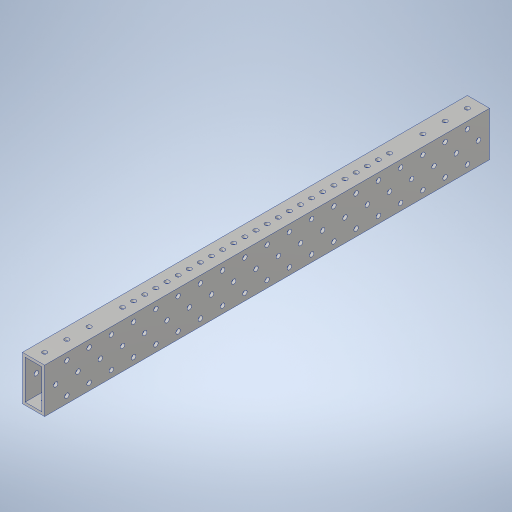
# Autodesk Inventor part: DB1-001
Saved by Autodesk Inventor 2023.4 (Build 274418000, 418)
## iProperties
RuleStatus: InUse
Created: 2025-01-07
Part Number: DB1-001
Material: Aluminum 6061
Document SubType Name: Modeling
Designer: mavericks
Mass: 304.185 g
Surface Area: 718.547 cm^2
Volume: 112.661 cm^3
Density: 2.7 g/cm^3
Appearance: Aluminum - Flat
AfterDocNew0: SHOW
AfterDocOpen0: SHOW
Author: mavericks
Autodesk Inventor part; units mm, degrees
ref_plane "YZ Plane" through (0, 0, 0) normal (1, 0, 0) x (0, 1, 0)
ref_plane "XZ Plane" through (0, 0, 0) normal (0, 1, 0) x (-1, 0, 0)
ref_plane "XY Plane" through (0, 0, 0) normal (0, 0, 1) x (1, 0, 0)
sketch "Sketch1" plane through (0, 0, 0) normal (0, 0, 1) x (1, 0, 0)
  line L0 (-12.7, -25.4) -> (12.7, -25.4)
  line L1 (12.7, -25.4) -> (12.7, 25.4)
  line L2 (12.7, 25.4) -> (-12.7, 25.4)
  line L3 (-12.7, 25.4) -> (-12.7, -25.4)
  line L4 (-12.7, -25.4) -> (12.7, 25.4) construction
  line L5 (12.7, -25.4) -> (-12.7, 25.4) construction
  line L6 (-9.525, 22.225) -> (9.525, 22.225)
  line L7 (9.525, 22.225) -> (9.525, -22.225)
  line L8 (9.525, -22.225) -> (-9.525, -22.225)
  line L9 (-9.525, -22.225) -> (-9.525, 22.225)
  point P0 (0, 0)
  dimension "width" = 25.4
  dimension "height" = 50.8
  dimension "thickness" = 3.175
  constraints: 20 end point, 4 parallel, 2 midpoint, 2 perpendicular, 1 horizontal, 3 other
  measures "width" distance of L2.end L1.end
  measures "height" distance of L1.end L0.end
  measures "thickness" distance between parallel lines of L2 L6
extrude "Extrusion1" add sketch "Sketch1" along normal mid plane 508
sketch "Sketch2" plane through (-12.7, 25.4, 254) normal (0, 1, 0) x (1, 0, 0)
  line L0 (25.4, 0) -> (0, 0) projected
  line L1 (12.7, 254) -> (0, 254) construction
  line L2 (0, 0) -> (0, 508) projected
  line L3 (12.7, 266.7) -> (12.7, 241.3) construction
  line L4 (12.7, 254) -> (12.7, 228.6) construction
  line L5 (12.7, 241.3) -> (12.7, 215.9) construction
  line L6 (12.7, 228.6) -> (12.7, 203.2) construction
  line L7 (12.7, 215.9) -> (12.7, 190.5) construction
  line L8 (12.7, 203.2) -> (12.7, 177.8) construction
  line L9 (12.7, 190.5) -> (12.7, 165.1) construction
  line L10 (12.7, 177.8) -> (12.7, 152.4) construction
  line L11 (12.7, 165.1) -> (12.7, 139.7) construction
  line L12 (12.7, 152.4) -> (12.7, 127) construction
  line L13 (12.7, 139.7) -> (12.7, 114.3) construction
  line L14 (12.7, 127) -> (12.7, 101.6) construction
  point P0 (12.7, 12.7)
  point P1 (12.7, 38.1)
  point P2 (12.7, 63.5)
  point P3 (12.7, 0)
  point P4 (12.7, 0)
  point P5 (12.7, 495.3)
  point P6 (12.7, 469.9)
  point P7 (12.7, 444.5)
  point P8 (12.7, 279.4)
  point P9 (12.7, 292.1)
  point P10 (12.7, 304.8)
  point P11 (12.7, 317.5)
  point P12 (12.7, 330.2)
  point P13 (12.7, 342.9)
  point P14 (12.7, 355.6)
  point P15 (12.7, 368.3)
  point P16 (12.7, 381)
  point P17 (12.7, 393.7)
  point P18 (12.7, 406.4)
  point P19 (12.7, 114.3)
  dimension "d5" = 12.7
  dimension "d6" = 25.4
  dimension "d7" = 25.4
  dimension "d8" = 25.4
  dimension "d11" = 12.7
  dimension "d18" = 12.7
  constraints: 26 end point, 4 midpoint, 4 vertical alignment, 3 symmetric about line, 3 vertical, 1 coincident, 55 other
  measures "d5" distance of point (12.7, 0) point (12.7, 12.7)
  measures "d6" distance of point (12.7, 38.1) point (12.7, 12.7)
  measures "d7" distance of point (12.7, 63.5) point (12.7, 38.1)
  measures "d8" distance of L3.end L3.start
  measures "d11" distance of L3.start point (12.7, 279.4)
  measures "d18" distance of L3.end L4.end
hole "Hole1" at (0, 25.4, 241.3) at (0, 25.4, 215.9) at (0, 25.4, 190.5) at (0, 25.4, -241.3) at (0, 25.4, -215.9) at (0, 25.4, -190.5) at (0, 25.4, -12.7) at (0, 25.4, 12.7) at (0, 25.4, -25.4) at (0, 25.4, -38.1) at (0, 25.4, -50.8) at (0, 25.4, -63.5) at (0, 25.4, -76.2) at (0, 25.4, -88.9) at (0, 25.4, -101.6) at (0, 25.4, -114.3) at (0, 25.4, -127) at (0, 25.4, -139.7) at (0, 25.4, -152.4) at (0, 25.4, 25.4) at (0, 25.4, 0) at (0, 25.4, 38.1) at (0, 25.4, 50.8) at (0, 25.4, 63.5) at (0, 25.4, 76.2) at (0, 25.4, 88.9) at (0, 25.4, 101.6) at (0, 25.4, 114.3) at (0, 25.4, 127) at (0, 25.4, 139.7) at (0, 25.4, 152.4) direction (0, -1, 0) diameter 5.1054 end through all clearance for "Flat Head Machine Screw (82)" size "#10" standard "Ansi Unified Screw Threads"
sketch "Sketch3" plane through (12.7, -25.4, 254) normal (1, 0, 0) x (0, 0, -1)
  line L0 (0, 0) -> (0, 50.8) construction
  circle A0 centre (254, 42.8625) radius 4.7625 construction
  line L1 (0, 47.625) -> (508, 47.625) construction
  line L2 (508, 50.8) -> (0, 50.8) construction
  line L3 (0, 0) -> (0, 50.8) construction
  line L4 (508, 0) -> (0, 0) construction
  line L5 (508, 50.8) -> (508, 0) construction
  line L6 (254, 42.8625) -> (254, 7.9375) construction
  circle A1 centre (254, 7.9375) radius 4.7625 construction
  line L7 (0, 3.175) -> (508, 3.175) construction
  point P0 (254, 25.4)
  point P1 (266.7, 25.4)
  point P2 (254, 25.4)
  point P3 (241.3, 25.4)
  point P4 (228.6, 42.8625)
  point P5 (215.9, 25.4)
  point P6 (228.6, 7.9375)
  point P7 (203.2, 42.8625)
  point P8 (190.5, 25.4)
  point P9 (203.2, 7.9375)
  point P10 (177.8, 42.8625)
  point P11 (165.1, 25.4)
  point P12 (177.8, 7.9375)
  point P13 (152.4, 42.8625)
  point P14 (139.7, 25.4)
  point P15 (152.4, 7.9375)
  point P16 (127, 42.8625)
  point P17 (114.3, 25.4)
  point P18 (127, 7.9375)
  point P19 (101.6, 42.8625)
  point P20 (88.9, 25.4)
  point P21 (101.6, 7.9375)
  point P22 (76.2, 42.8625)
  point P23 (63.5, 25.4)
  point P24 (76.2, 7.9375)
  point P25 (50.8, 42.8625)
  point P26 (38.1, 25.4)
  point P27 (50.8, 7.9375)
  point P28 (25.4, 42.8625)
  point P29 (12.7, 25.4)
  point P30 (25.4, 7.9375)
  point P31 (279.4, 42.8625)
  point P32 (292.1, 25.4)
  point P33 (279.4, 7.9375)
  point P34 (304.8, 42.8625)
  point P35 (317.5, 25.4)
  point P36 (304.8, 7.9375)
  point P37 (330.2, 42.8625)
  point P38 (342.9, 25.4)
  point P39 (330.2, 7.9375)
  point P40 (355.6, 42.8625)
  point P41 (368.3, 25.4)
  point P42 (355.6, 7.9375)
  point P43 (381, 42.8625)
  point P44 (393.7, 25.4)
  point P45 (381, 7.9375)
  point P46 (406.4, 42.8625)
  point P47 (419.1, 25.4)
  point P48 (406.4, 7.9375)
  point P49 (431.8, 42.8625)
  point P50 (444.5, 25.4)
  point P51 (431.8, 7.9375)
  point P52 (457.2, 42.8625)
  point P53 (469.9, 25.4)
  point P54 (457.2, 7.9375)
  point P55 (482.6, 42.8625)
  point P56 (495.3, 25.4)
  point P57 (482.6, 7.9375)
  dimension "d31" = 12.7
  dimension "d33" = 9.525
  dimension "d34" = 9.525
  dimension "d35" = 12.7
  dimension "d38" = 25.4
  dimension "d45" = 25.4
  constraints: 5 coincident, 2 centre point, 2 end point, 2 horizontal, 2 horizontal alignment, 2 tangent, 1 midpoint, 1 vertical, 54 other
  measures "d31" horizontal distance of point (266.7, 25.4) point (254, 42.863)
  measures "d33" diameter of A0
  measures "d34" diameter of A1
  measures "d35" distance of point (254, 25.4) point (241.3, 25.4)
  measures "d38" distance of L6.start point (228.6, 42.863)
  measures "d45" distance of point (254, 42.863) point (279.4, 42.863)
hole "Hole2" at (12.7, 17.4625, 0) at (12.7, 0, -12.7) at (12.7, 0, 12.7) at (12.7, 0, 38.1) at (12.7, 0, 63.5) at (12.7, 0, 88.9) at (12.7, 0, 114.3) at (12.7, 0, 139.7) at (12.7, 0, 165.1) at (12.7, 0, 190.5) at (12.7, 0, 215.9) at (12.7, 0, 241.3) at (12.7, 17.4625, -25.4) at (12.7, 0, -38.1) at (12.7, 17.4625, -50.8) at (12.7, 0, -63.5) at (12.7, 17.4625, -76.2) at (12.7, 0, -88.9) at (12.7, 17.4625, -101.6) at (12.7, 0, -114.3) at (12.7, 17.4625, -127) at (12.7, 0, -139.7) at (12.7, 17.4625, -152.4) at (12.7, 0, -165.1) at (12.7, 17.4625, -177.8) at (12.7, 0, -190.5) at (12.7, 17.4625, -203.2) at (12.7, 0, -215.9) at (12.7, 17.4625, -228.6) at (12.7, 0, -241.3) at (12.7, 17.4625, 228.6) at (12.7, 17.4625, 203.2) at (12.7, 17.4625, 177.8) at (12.7, 17.4625, 152.4) at (12.7, 17.4625, 127) at (12.7, 17.4625, 101.6) at (12.7, 17.4625, 76.2) at (12.7, 17.4625, 50.8) at (12.7, 17.4625, 25.4) at (12.7, -17.4625, -50.8) at (12.7, -17.4625, -76.2) at (12.7, -17.4625, -101.6) at (12.7, -17.4625, -127) at (12.7, -17.4625, -152.4) at (12.7, -17.4625, -177.8) at (12.7, -17.4625, -203.2) at (12.7, -17.4625, -228.6) at (12.7, -17.4625, -25.4) at (12.7, -17.4625, 0) at (12.7, -17.4625, 25.4) direction (-1, 0, 0) diameter 5.1054 end through all and at (12.7, -17.4625, 50.8) (12.7, -17.4625, 76.2) (12.7, -17.4625, 101.6) (12.7, -17.4625, 127) (12.7, -17.4625, 152.4) (12.7, -17.4625, 177.8) (12.7, -17.4625, 203.2) (12.7, -17.4625, 228.6) clearance for "Flat Head Machine Screw (82)" size "#10" standard "Ansi Unified Screw Threads"
equation "\"d7\" = d6"
body "Solid1"
